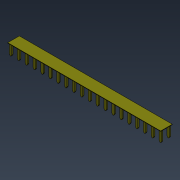
# Autodesk Inventor part: SSW-120-01-F-D_pin
Saved by Autodesk Inventor 2022.1 (Build 261234020, 234B)
## iProperties
Created: 2015-08-09
Part Number: SSW-120-01-F-D_pin
Catalog Web Link: www.cadenas.de
Description: SSW Series Pin-SSW Series - (2,54 mm) .100" Surface Mount Terminal & Through-Hole .025" Square Post Socket
Vendor: SAMTEC
Document SubType Name: Modeling
Designer: PARTuser1
Manufacturer: SAMTEC
Mass: 0.0669125 g
Surface Area: 7.06347 cm^2
Volume: 0.0669125 cm^3
Density: 1 g/cm^3
Material: Allgemein
Appearance: PSOLRGB-255-255-0
Category: PARTsolutions
Company: SAMTEC
PSOL_IDENT_0: {$CADENAS_DATA\23d-libs\samtec\modelling\ssw\parts\ssw_pin.prj},220 {VTYP=3D},{NB=SSW-120-01-F-D_pin
PSOL_IDENT_1: },{LINA=SSW-120-01-F-D_pin},{NN=SSW Series Pin},{DATE=19.06.2015 09:33:41},{GEOMDATE=19.06.2015 09:3
PSOL_IDENT_2: 3:00},{VERSION=},{LINEID=10},{LINESUBID=-1},{WBVAR=POS,LS,PLOPT,ROW,TOPT,POLOPT,LLOPT}  {NB=SSW-120-
PSOL_IDENT_3: 01-F-D_pin},{LINA=SSW-120-01-F-D_pin},{KT=DUMMY},{PN=SSW-120-01-F-D},{SERIES=SSW},{POS=20},{POSATOF=
PSOL_IDENT_4: 20},{LS=01},{LSALG= '01','-01','02','-02','03','-03','04','-04','06','-06','21','-21','22','-22','23'
PSOL_IDENT_5: ,'-23','24','-24' },{PLOPT=F},{PLOPTALG= 'G','-G - Gold, 20micro\" Au / 50micro\" Ni Min on Contact,
PSOL_IDENT_6: 3micro\" Au / 50micro\" Ni Min on Tail','S','-S - Selective, 30micro\" Au / 50micro\" Ni Min on Con
PSOL_IDENT_7: tact, Matte Tin Tail','H','-H - Heavy Gold 30micro\" Au / 50micro\" Ni Min on Contact, 3micro\" Au /
PSOL_IDENT_8: 50micro\" Ni Min on Tail' ,'F','-F - Flash Selective, 3micro\" Au / 50micro\" Ni Min on Contact, Ma
PSOL_IDENT_9: tte Tin Tail','STL','-STL - Selective, 30micro\" Au / 50micro\" Ni Min on Contact Area, Tin/Lead (90
PSOL_IDENT_10: /10 +/-5%) Tail','SM','-SM - Selective, 30micro\" Au / 50micro\" Ni Min on Contact, Matte Tin Tail','
PSOL_IDENT_11: FM','-FM - Flash Selective, 3micro\" Au / 50micro\" Ni Min on Contact, Matte Tin Tail','L','-L - Lig
PSOL_IDENT_12: ht Selective, 10micro\" Au / 50micro\" Ni Min on Contact Area, Matte Tin Tail','T','-T - Matte Tin C
PSOL_IDENT_13: ontact and Tail','E','-E - 50micro\" Extra Heavy Gold in Contact Area, 3micro\" Gold on Tail','TL','
PSOL_IDENT_14: -TL - Tin/Lead (90/10 ± 5%) Contact and Tail','TM','-TM - Matte Tin Contact and Tail' },{ROW=D},{ROW
PSOL_IDENT_15: ALG= 'S','-S - Single','D','-D - Double','T','-T - Triple', 'P','-P - Single Notched','Q','-Q - Trip
PSOL_IDENT_16: le with only Outer 2 Rows Filled' },{TOPT=},{TOPTALG= '','Straight' },{TOPTPN=},{POLOPT=},{POLOPTALG=
PSOL_IDENT_17: '','Not Selected','001','001','002','002','003','003','004','004','005','005','006','006','007','00
PSOL_IDENT_18: 7','008','008','009','009','010','010','011','011','012','012','013','013','014','014','015','015','
PSOL_IDENT_19: 016','016','017','017','018','018','019','019','020','020','021','021','022','022','023','023','024'
PSOL_IDENT_20: ,'024','025','025','026','026','027','027','028','028','029','029','030','030','031','031','032','03
PSOL_IDENT_21: 2','033','033','034','034','035','035','036','036','037','037','038','038','039','039','040','040' }
PSOL_IDENT_22: ,{POLOPTMAX=480},{POLOPTMAX2='001','001','002','002','003','003','004','004','005','005','006','006'
PSOL_IDENT_23: ,'007','007','008','008','009','009','010','010','011','011','012','012','013','013','014','014','01
PSOL_IDENT_24: 5','015','016','016','017','017','018','018','019','019','020','020','021','021','022','022','023','
PSOL_IDENT_25: 023','024','024','025','025','026','026','027','027','028','028','029','029','030','030','031','031'
PSOL_IDENT_26: ,'032','032','033','033','034','034','035','035','036','036','037','037','038','038','039','039','04
PSOL_IDENT_27: 0','040'},{POLARIZE='001','001','002','002','003','003','004','004','005','005','006','006','007','0
PSOL_IDENT_28: 07','008','008','009','009','010','010','011','011','012','012','013','013','014','014','015','015','
PSOL_IDENT_29: 016','016','017','017','018','018','019','019','020','020','021','021','022','022','023','023','024'
PSOL_IDENT_30: ,'024','025','025','026','026','027','027','028','028','029','029','030','030','031','031','032','03
PSOL_IDENT_31: 2','033','033','034','034','035','035','036','036','037','037','038','038','039','039','040','040','
PSOL_IDENT_32: 041','041','042','042','043','043','044','044','045','045','046','046','047','047','048','048','049'
PSOL_IDENT_33: ,'049','050','050','051','051','052','052','053','053','054','054','055','055','056','056','057','05
PSOL_IDENT_34: 7','058','058','059','059','060','060','061','061','062','062','063','063','064','064','065','065','
PSOL_IDENT_35: 066','066','067','067','068','068','069','069','070','070','071','071','072','072','073','073','074'
PSOL_IDENT_36: ,'074','075','075','076','076','077','077','078','078','079','079','080','080','081','081','082','08
PSOL_IDENT_37: 2','083','083','084','084','085','085','086','086','087','087','088','088','089','089','090','090','
PSOL_IDENT_38: 091','091','092','092','093','093','094','094','095','095','096','096','097','097','098','098','099'
PSOL_IDENT_39: ,'099','100','100','101','101','102','102','103','103','104','104','105','105','106','106','107','10
PSOL_IDENT_40: 7','108','108','109','109','110','110','111','111','112','112','113','113','114','114','115','115','
PSOL_IDENT_41: 116','116','117','117','118','118','119','119','120','120','121','121','122','122','123','123','124'
PSOL_IDENT_42: ,'124','125','125','126','126','127','127','128','128','129','129','130','130','131','131','132','13
PSOL_IDENT_43: 2','133','133','134','134','135','135','136','136','137','137','138','138','139','139','140','140','
PSOL_IDENT_44: 141','141','142','142','143','143','144','144','145','145','146','146','147','147','148','148','149'
PSOL_IDENT_45: ,'149','150','150'},{POLOPTPN=},{LLOPT=},{LLOPTALG= '','Not Selected','LL','-LL - Locking Lead' },{L
PSOL_IDENT_46: LOPTPN=},{B=0.104},{C=0.000},{R=2.020},{OEN=2}
NN: SSW Series Pin
NT: SSW Series - (2,54 mm) .100" Surface Mount Terminal & Through-Hole .025" Square Post Socket
NB: SSW-120-01-F-D_pin
NBSYN: $PN._pin
LINA: SSW-120-01-F-D_pin
SERIES: SSW
POS: -20
LS: -01
PLOPT: -F - Flash Selective, 3micro" Au / 50micro" Ni Min on Contact, Matte Tin Tail
ROW: -D - Double
TOPT: Straight
POLOPT: Not Selected
LLOPT: Not Selected
SUPPLIER: SAMTEC
ARTICLENO: SSW-120-01-F-D_pin
BOMINFO: SSW-120-01-F-D_pin
CREATOR: CADENAS GmbH
Title: SSW-120-01-F-D_pin
Author: Cadenas PARTsolutions
Comments: SSW Series - (2,54 mm) .100" Surface Mount Terminal & Through-Hole .025" Square Post Socket
Autodesk Inventor part; units mm, degrees
sketch "Sketch_2" plane through (0, 0, 0) normal (1, 0, 0) x (0, 1, 0)
  line L0 (3.6576, 1.4732) -> (0, 1.4732)
  line L1 (0, 1.4732) -> (0, 1.0668)
  line L2 (0, 1.0668) -> (3.5306, 1.0668)
  line L3 (3.5306, 1.0668) -> (3.5306, -1.0668)
  line L4 (3.5306, -1.0668) -> (0, -1.0668)
  line L5 (0, -1.0668) -> (0, -1.4732)
  line L6 (0, -1.4732) -> (3.6576, -1.4732)
  line L7 (3.6576, -1.4732) -> (3.6576, 1.4732)
  constraints: 16 end point
extrude "Extrusion1" add sketch "Sketch_2" along normal mid plane 49.3014
sketch "Sketch_13" plane through (0, 3.5306, 0) normal (0, 1, 0) x (1, 0, 0)
  line L0 (-24.6507, 1.8796) -> (-24.6507, -1.8796)
  line L1 (-24.6507, -1.8796) -> (24.6507, -1.8796)
  line L2 (24.6507, -1.8796) -> (24.6507, 1.8796)
  line L3 (24.6507, 1.8796) -> (-24.6507, 1.8796)
  constraints: 8 end point
extrude "Extrusion2" add sketch "Sketch_13" along normal blind 0.127
sketch "Sketch_8" plane through (0, 0, 0) normal (0, 0, 1) x (1, 0, 0)
  line L0 (-26.2763, -21.8694) -> (99.9363, -21.8694)
  line L1 (99.9363, -21.8694) -> (99.9363, 3.5306)
  line L2 (99.9363, 3.5306) -> (98.1837, 3.5306)
  line L3 (98.1837, 3.5306) -> (98.1837, -8.89)
  line L4 (98.1837, -8.89) -> (97.3963, -8.89)
  line L5 (97.3963, -8.89) -> (97.3963, 3.5306)
  line L6 (97.3963, 3.5306) -> (95.6437, 3.5306)
  line L7 (95.6437, 3.5306) -> (95.6437, -8.89)
  line L8 (95.6437, -8.89) -> (94.8563, -8.89)
  line L9 (94.8563, -8.89) -> (94.8563, 3.5306)
  line L10 (94.8563, 3.5306) -> (93.1037, 3.5306)
  line L11 (93.1037, 3.5306) -> (93.1037, -8.89)
  line L12 (93.1037, -8.89) -> (92.3163, -8.89)
  line L13 (92.3163, -8.89) -> (92.3163, 3.5306)
  line L14 (92.3163, 3.5306) -> (90.5637, 3.5306)
  line L15 (90.5637, 3.5306) -> (90.5637, -8.89)
  line L16 (90.5637, -8.89) -> (89.7763, -8.89)
  line L17 (89.7763, -8.89) -> (89.7763, 3.5306)
  line L18 (89.7763, 3.5306) -> (88.0237, 3.5306)
  line L19 (88.0237, 3.5306) -> (88.0237, -8.89)
  line L20 (88.0237, -8.89) -> (87.2363, -8.89)
  line L21 (87.2363, -8.89) -> (87.2363, 3.5306)
  line L22 (87.2363, 3.5306) -> (85.4837, 3.5306)
  line L23 (85.4837, 3.5306) -> (85.4837, -8.89)
  line L24 (85.4837, -8.89) -> (84.6963, -8.89)
  line L25 (84.6963, -8.89) -> (84.6963, 3.5306)
  line L26 (84.6963, 3.5306) -> (82.9437, 3.5306)
  line L27 (82.9437, 3.5306) -> (82.9437, -8.89)
  line L28 (82.9437, -8.89) -> (82.1563, -8.89)
  line L29 (82.1563, -8.89) -> (82.1563, 3.5306)
  line L30 (82.1563, 3.5306) -> (80.4037, 3.5306)
  line L31 (80.4037, 3.5306) -> (80.4037, -8.89)
  line L32 (80.4037, -8.89) -> (79.6163, -8.89)
  line L33 (79.6163, -8.89) -> (79.6163, 3.5306)
  line L34 (79.6163, 3.5306) -> (77.8637, 3.5306)
  line L35 (77.8637, 3.5306) -> (77.8637, -8.89)
  line L36 (77.8637, -8.89) -> (77.0763, -8.89)
  line L37 (77.0763, -8.89) -> (77.0763, 3.5306)
  line L38 (77.0763, 3.5306) -> (75.3237, 3.5306)
  line L39 (75.3237, 3.5306) -> (75.3237, -8.89)
  line L40 (75.3237, -8.89) -> (74.5363, -8.89)
  line L41 (74.5363, -8.89) -> (74.5363, 3.5306)
  line L42 (74.5363, 3.5306) -> (72.7837, 3.5306)
  line L43 (72.7837, 3.5306) -> (72.7837, -8.89)
  line L44 (72.7837, -8.89) -> (71.9963, -8.89)
  line L45 (71.9963, -8.89) -> (71.9963, 3.5306)
  line L46 (71.9963, 3.5306) -> (70.2437, 3.5306)
  line L47 (70.2437, 3.5306) -> (70.2437, -8.89)
  line L48 (70.2437, -8.89) -> (69.4563, -8.89)
  line L49 (69.4563, -8.89) -> (69.4563, 3.5306)
  line L50 (69.4563, 3.5306) -> (67.7037, 3.5306)
  line L51 (67.7037, 3.5306) -> (67.7037, -8.89)
  line L52 (67.7037, -8.89) -> (66.9163, -8.89)
  line L53 (66.9163, -8.89) -> (66.9163, 3.5306)
  line L54 (66.9163, 3.5306) -> (65.1637, 3.5306)
  line L55 (65.1637, 3.5306) -> (65.1637, -8.89)
  line L56 (65.1637, -8.89) -> (64.3763, -8.89)
  line L57 (64.3763, -8.89) -> (64.3763, 3.5306)
  line L58 (64.3763, 3.5306) -> (62.6237, 3.5306)
  line L59 (62.6237, 3.5306) -> (62.6237, -8.89)
  line L60 (62.6237, -8.89) -> (61.8363, -8.89)
  line L61 (61.8363, -8.89) -> (61.8363, 3.5306)
  line L62 (61.8363, 3.5306) -> (60.0837, 3.5306)
  line L63 (60.0837, 3.5306) -> (60.0837, -8.89)
  line L64 (60.0837, -8.89) -> (59.2963, -8.89)
  line L65 (59.2963, -8.89) -> (59.2963, 3.5306)
  line L66 (59.2963, 3.5306) -> (57.5437, 3.5306)
  line L67 (57.5437, 3.5306) -> (57.5437, -8.89)
  line L68 (57.5437, -8.89) -> (56.7563, -8.89)
  line L69 (56.7563, -8.89) -> (56.7563, 3.5306)
  line L70 (56.7563, 3.5306) -> (55.0037, 3.5306)
  line L71 (55.0037, 3.5306) -> (55.0037, -8.89)
  line L72 (55.0037, -8.89) -> (54.2163, -8.89)
  line L73 (54.2163, -8.89) -> (54.2163, 3.5306)
  line L74 (54.2163, 3.5306) -> (52.4637, 3.5306)
  line L75 (52.4637, 3.5306) -> (52.4637, -8.89)
  line L76 (52.4637, -8.89) -> (51.6763, -8.89)
  line L77 (51.6763, -8.89) -> (51.6763, 3.5306)
  line L78 (51.6763, 3.5306) -> (49.9237, 3.5306)
  line L79 (49.9237, 3.5306) -> (49.9237, -8.89)
  line L80 (49.9237, -8.89) -> (49.1363, -8.89)
  line L81 (49.1363, -8.89) -> (49.1363, 3.5306)
  line L82 (49.1363, 3.5306) -> (47.3837, 3.5306)
  line L83 (47.3837, 3.5306) -> (47.3837, -8.89)
  line L84 (47.3837, -8.89) -> (46.5963, -8.89)
  line L85 (46.5963, -8.89) -> (46.5963, 3.5306)
  line L86 (46.5963, 3.5306) -> (44.8437, 3.5306)
  line L87 (44.8437, 3.5306) -> (44.8437, -8.89)
  line L88 (44.8437, -8.89) -> (44.0563, -8.89)
  line L89 (44.0563, -8.89) -> (44.0563, 3.5306)
  line L90 (44.0563, 3.5306) -> (42.3037, 3.5306)
  line L91 (42.3037, 3.5306) -> (42.3037, -8.89)
  line L92 (42.3037, -8.89) -> (41.5163, -8.89)
  line L93 (41.5163, -8.89) -> (41.5163, 3.5306)
  line L94 (41.5163, 3.5306) -> (39.7637, 3.5306)
  line L95 (39.7637, 3.5306) -> (39.7637, -8.89)
  line L96 (39.7637, -8.89) -> (38.9763, -8.89)
  line L97 (38.9763, -8.89) -> (38.9763, 3.5306)
  line L98 (38.9763, 3.5306) -> (37.2237, 3.5306)
  line L99 (37.2237, 3.5306) -> (37.2237, -8.89)
  line L100 (37.2237, -8.89) -> (36.4363, -8.89)
  line L101 (36.4363, -8.89) -> (36.4363, 3.5306)
  line L102 (36.4363, 3.5306) -> (34.6837, 3.5306)
  line L103 (34.6837, 3.5306) -> (34.6837, -8.89)
  line L104 (34.6837, -8.89) -> (33.8963, -8.89)
  line L105 (33.8963, -8.89) -> (33.8963, 3.5306)
  line L106 (33.8963, 3.5306) -> (32.1437, 3.5306)
  line L107 (32.1437, 3.5306) -> (32.1437, -8.89)
  line L108 (32.1437, -8.89) -> (31.3563, -8.89)
  line L109 (31.3563, -8.89) -> (31.3563, 3.5306)
  line L110 (31.3563, 3.5306) -> (29.6037, 3.5306)
  line L111 (29.6037, 3.5306) -> (29.6037, -8.89)
  line L112 (29.6037, -8.89) -> (28.8163, -8.89)
  line L113 (28.8163, -8.89) -> (28.8163, 3.5306)
  line L114 (28.8163, 3.5306) -> (27.0637, 3.5306)
  line L115 (27.0637, 3.5306) -> (27.0637, -8.89)
  line L116 (27.0637, -8.89) -> (26.2763, -8.89)
  line L117 (26.2763, -8.89) -> (26.2763, 3.5306)
  line L118 (26.2763, 3.5306) -> (24.5237, 3.5306)
  line L119 (24.5237, 3.5306) -> (24.5237, -8.89)
  line L120 (24.5237, -8.89) -> (23.7363, -8.89)
  line L121 (23.7363, -8.89) -> (23.7363, 3.5306)
  line L122 (23.7363, 3.5306) -> (21.9837, 3.5306)
  line L123 (21.9837, 3.5306) -> (21.9837, -8.89)
  line L124 (21.9837, -8.89) -> (21.1963, -8.89)
  line L125 (21.1963, -8.89) -> (21.1963, 3.5306)
  line L126 (21.1963, 3.5306) -> (19.4437, 3.5306)
  line L127 (19.4437, 3.5306) -> (19.4437, -8.89)
  line L128 (19.4437, -8.89) -> (18.6563, -8.89)
  line L129 (18.6563, -8.89) -> (18.6563, 3.5306)
  line L130 (18.6563, 3.5306) -> (16.9037, 3.5306)
  line L131 (16.9037, 3.5306) -> (16.9037, -8.89)
  line L132 (16.9037, -8.89) -> (16.1163, -8.89)
  line L133 (16.1163, -8.89) -> (16.1163, 3.5306)
  line L134 (16.1163, 3.5306) -> (14.3637, 3.5306)
  line L135 (14.3637, 3.5306) -> (14.3637, -8.89)
  line L136 (14.3637, -8.89) -> (13.5763, -8.89)
  line L137 (13.5763, -8.89) -> (13.5763, 3.5306)
  line L138 (13.5763, 3.5306) -> (11.8237, 3.5306)
  line L139 (11.8237, 3.5306) -> (11.8237, -8.89)
  line L140 (11.8237, -8.89) -> (11.0363, -8.89)
  line L141 (11.0363, -8.89) -> (11.0363, 3.5306)
  line L142 (11.0363, 3.5306) -> (9.2837, 3.5306)
  line L143 (9.2837, 3.5306) -> (9.2837, -8.89)
  line L144 (9.2837, -8.89) -> (8.4963, -8.89)
  line L145 (8.4963, -8.89) -> (8.4963, 3.5306)
  line L146 (8.4963, 3.5306) -> (6.7437, 3.5306)
  line L147 (6.7437, 3.5306) -> (6.7437, -8.89)
  line L148 (6.7437, -8.89) -> (5.9563, -8.89)
  line L149 (5.9563, -8.89) -> (5.9563, 3.5306)
  line L150 (5.9563, 3.5306) -> (4.2037, 3.5306)
  line L151 (4.2037, 3.5306) -> (4.2037, -8.89)
  line L152 (4.2037, -8.89) -> (3.4163, -8.89)
  line L153 (3.4163, -8.89) -> (3.4163, 3.5306)
  line L154 (3.4163, 3.5306) -> (1.6637, 3.5306)
  line L155 (1.6637, 3.5306) -> (1.6637, -8.89)
  line L156 (1.6637, -8.89) -> (0.8763, -8.89)
  line L157 (0.8763, -8.89) -> (0.8763, 3.5306)
  line L158 (0.8763, 3.5306) -> (-0.8763, 3.5306)
  line L159 (-0.8763, 3.5306) -> (-0.8763, -8.89)
  line L160 (-0.8763, -8.89) -> (-1.6637, -8.89)
  line L161 (-1.6637, -8.89) -> (-1.6637, 3.5306)
  line L162 (-1.6637, 3.5306) -> (-3.4163, 3.5306)
  line L163 (-3.4163, 3.5306) -> (-3.4163, -8.89)
  line L164 (-3.4163, -8.89) -> (-4.2037, -8.89)
  line L165 (-4.2037, -8.89) -> (-4.2037, 3.5306)
  line L166 (-4.2037, 3.5306) -> (-5.9563, 3.5306)
  line L167 (-5.9563, 3.5306) -> (-5.9563, -8.89)
  line L168 (-5.9563, -8.89) -> (-6.7437, -8.89)
  line L169 (-6.7437, -8.89) -> (-6.7437, 3.5306)
  line L170 (-6.7437, 3.5306) -> (-8.4963, 3.5306)
  line L171 (-8.4963, 3.5306) -> (-8.4963, -8.89)
  line L172 (-8.4963, -8.89) -> (-9.2837, -8.89)
  line L173 (-9.2837, -8.89) -> (-9.2837, 3.5306)
  line L174 (-9.2837, 3.5306) -> (-11.0363, 3.5306)
  line L175 (-11.0363, 3.5306) -> (-11.0363, -8.89)
  line L176 (-11.0363, -8.89) -> (-11.8237, -8.89)
  line L177 (-11.8237, -8.89) -> (-11.8237, 3.5306)
  line L178 (-11.8237, 3.5306) -> (-13.5763, 3.5306)
  line L179 (-13.5763, 3.5306) -> (-13.5763, -8.89)
  line L180 (-13.5763, -8.89) -> (-14.3637, -8.89)
  line L181 (-14.3637, -8.89) -> (-14.3637, 3.5306)
  line L182 (-14.3637, 3.5306) -> (-16.1163, 3.5306)
  line L183 (-16.1163, 3.5306) -> (-16.1163, -8.89)
  line L184 (-16.1163, -8.89) -> (-16.9037, -8.89)
  line L185 (-16.9037, -8.89) -> (-16.9037, 3.5306)
  line L186 (-16.9037, 3.5306) -> (-18.6563, 3.5306)
  line L187 (-18.6563, 3.5306) -> (-18.6563, -8.89)
  line L188 (-18.6563, -8.89) -> (-19.4437, -8.89)
  line L189 (-19.4437, -8.89) -> (-19.4437, 3.5306)
  line L190 (-19.4437, 3.5306) -> (-21.1963, 3.5306)
  line L191 (-21.1963, 3.5306) -> (-21.1963, -8.89)
  line L192 (-21.1963, -8.89) -> (-21.9837, -8.89)
  line L193 (-21.9837, -8.89) -> (-21.9837, 3.5306)
  line L194 (-21.9837, 3.5306) -> (-23.7363, 3.5306)
  line L195 (-23.7363, 3.5306) -> (-23.7363, -8.89)
  line L196 (-23.7363, -8.89) -> (-24.5237, -8.89)
  line L197 (-24.5237, -8.89) -> (-24.5237, 3.5306)
  line L198 (-24.5237, 3.5306) -> (-26.2763, 3.5306)
  line L199 (-26.2763, 3.5306) -> (-26.2763, -21.8694)
  constraints: 400 end point
extrude "Extrusion3" cut sketch "Sketch_8" along normal mid plane 50.8
sketch "Sketch_6" plane through (0, 0, 0) normal (0, 0, 1) x (1, 0, 0)
  line L0 (-24.5237, 0.4399) -> (-24.5237, -2.54)
  line L1 (-24.5237, -2.54) -> (24.5237, -2.54)
  line L2 (24.5237, -2.54) -> (24.5237, 0.4399)
  line L3 (24.5237, 0.4399) -> (24.2697, 0)
  line L4 (24.2697, 0) -> (23.9903, 0)
  line L5 (23.9903, 0) -> (23.7363, 0.4399)
  line L6 (23.7363, 0.4399) -> (23.7363, -2.032)
  line L7 (23.7363, -2.032) -> (21.9837, -2.032)
  line L8 (21.9837, -2.032) -> (21.9837, 0.4399)
  line L9 (21.9837, 0.4399) -> (21.7297, 0)
  line L10 (21.7297, 0) -> (21.4503, 0)
  line L11 (21.4503, 0) -> (21.1963, 0.4399)
  line L12 (21.1963, 0.4399) -> (21.1963, -2.032)
  line L13 (21.1963, -2.032) -> (19.4437, -2.032)
  line L14 (19.4437, -2.032) -> (19.4437, 0.4399)
  line L15 (19.4437, 0.4399) -> (19.1897, 0)
  line L16 (19.1897, 0) -> (18.9103, 0)
  line L17 (18.9103, 0) -> (18.6563, 0.4399)
  line L18 (18.6563, 0.4399) -> (18.6563, -2.032)
  line L19 (18.6563, -2.032) -> (16.9037, -2.032)
  line L20 (16.9037, -2.032) -> (16.9037, 0.4399)
  line L21 (16.9037, 0.4399) -> (16.6497, 0)
  line L22 (16.6497, 0) -> (16.3703, 0)
  line L23 (16.3703, 0) -> (16.1163, 0.4399)
  line L24 (16.1163, 0.4399) -> (16.1163, -2.032)
  line L25 (16.1163, -2.032) -> (14.3637, -2.032)
  line L26 (14.3637, -2.032) -> (14.3637, 0.4399)
  line L27 (14.3637, 0.4399) -> (14.1097, 0)
  line L28 (14.1097, 0) -> (13.8303, 0)
  line L29 (13.8303, 0) -> (13.5763, 0.4399)
  line L30 (13.5763, 0.4399) -> (13.5763, -2.032)
  line L31 (13.5763, -2.032) -> (11.8237, -2.032)
  line L32 (11.8237, -2.032) -> (11.8237, 0.4399)
  line L33 (11.8237, 0.4399) -> (11.5697, 0)
  line L34 (11.5697, 0) -> (11.2903, 0)
  line L35 (11.2903, 0) -> (11.0363, 0.4399)
  line L36 (11.0363, 0.4399) -> (11.0363, -2.032)
  line L37 (11.0363, -2.032) -> (9.2837, -2.032)
  line L38 (9.2837, -2.032) -> (9.2837, 0.4399)
  line L39 (9.2837, 0.4399) -> (9.0297, 0)
  line L40 (9.0297, 0) -> (8.7503, 0)
  line L41 (8.7503, 0) -> (8.4963, 0.4399)
  line L42 (8.4963, 0.4399) -> (8.4963, -2.032)
  line L43 (8.4963, -2.032) -> (6.7437, -2.032)
  line L44 (6.7437, -2.032) -> (6.7437, 0.4399)
  line L45 (6.7437, 0.4399) -> (6.4897, 0)
  line L46 (6.4897, 0) -> (6.2103, 0)
  line L47 (6.2103, 0) -> (5.9563, 0.4399)
  line L48 (5.9563, 0.4399) -> (5.9563, -2.032)
  line L49 (5.9563, -2.032) -> (4.2037, -2.032)
  line L50 (4.2037, -2.032) -> (4.2037, 0.4399)
  line L51 (4.2037, 0.4399) -> (3.9497, 0)
  line L52 (3.9497, 0) -> (3.6703, 0)
  line L53 (3.6703, 0) -> (3.4163, 0.4399)
  line L54 (3.4163, 0.4399) -> (3.4163, -2.032)
  line L55 (3.4163, -2.032) -> (1.6637, -2.032)
  line L56 (1.6637, -2.032) -> (1.6637, 0.4399)
  line L57 (1.6637, 0.4399) -> (1.4097, 0)
  line L58 (1.4097, 0) -> (1.1303, 0)
  line L59 (1.1303, 0) -> (0.8763, 0.4399)
  line L60 (0.8763, 0.4399) -> (0.8763, -2.032)
  line L61 (0.8763, -2.032) -> (-0.8763, -2.032)
  line L62 (-0.8763, -2.032) -> (-0.8763, 0.4399)
  line L63 (-0.8763, 0.4399) -> (-1.1303, 0)
  line L64 (-1.1303, 0) -> (-1.4097, 0)
  line L65 (-1.4097, 0) -> (-1.6637, 0.4399)
  line L66 (-1.6637, 0.4399) -> (-1.6637, -2.032)
  line L67 (-1.6637, -2.032) -> (-3.4163, -2.032)
  line L68 (-3.4163, -2.032) -> (-3.4163, 0.4399)
  line L69 (-3.4163, 0.4399) -> (-3.6703, 0)
  line L70 (-3.6703, 0) -> (-3.9497, 0)
  line L71 (-3.9497, 0) -> (-4.2037, 0.4399)
  line L72 (-4.2037, 0.4399) -> (-4.2037, -2.032)
  line L73 (-4.2037, -2.032) -> (-5.9563, -2.032)
  line L74 (-5.9563, -2.032) -> (-5.9563, 0.4399)
  line L75 (-5.9563, 0.4399) -> (-6.2103, 0)
  line L76 (-6.2103, 0) -> (-6.4897, 0)
  line L77 (-6.4897, 0) -> (-6.7437, 0.4399)
  line L78 (-6.7437, 0.4399) -> (-6.7437, -2.032)
  line L79 (-6.7437, -2.032) -> (-8.4963, -2.032)
  line L80 (-8.4963, -2.032) -> (-8.4963, 0.4399)
  line L81 (-8.4963, 0.4399) -> (-8.7503, 0)
  line L82 (-8.7503, 0) -> (-9.0297, 0)
  line L83 (-9.0297, 0) -> (-9.2837, 0.4399)
  line L84 (-9.2837, 0.4399) -> (-9.2837, -2.032)
  line L85 (-9.2837, -2.032) -> (-11.0363, -2.032)
  line L86 (-11.0363, -2.032) -> (-11.0363, 0.4399)
  line L87 (-11.0363, 0.4399) -> (-11.2903, 0)
  line L88 (-11.2903, 0) -> (-11.5697, 0)
  line L89 (-11.5697, 0) -> (-11.8237, 0.4399)
  line L90 (-11.8237, 0.4399) -> (-11.8237, -2.032)
  line L91 (-11.8237, -2.032) -> (-13.5763, -2.032)
  line L92 (-13.5763, -2.032) -> (-13.5763, 0.4399)
  line L93 (-13.5763, 0.4399) -> (-13.8303, 0)
  line L94 (-13.8303, 0) -> (-14.1097, 0)
  line L95 (-14.1097, 0) -> (-14.3637, 0.4399)
  line L96 (-14.3637, 0.4399) -> (-14.3637, -2.032)
  line L97 (-14.3637, -2.032) -> (-16.1163, -2.032)
  line L98 (-16.1163, -2.032) -> (-16.1163, 0.4399)
  line L99 (-16.1163, 0.4399) -> (-16.3703, 0)
  line L100 (-16.3703, 0) -> (-16.6497, 0)
  line L101 (-16.6497, 0) -> (-16.9037, 0.4399)
  line L102 (-16.9037, 0.4399) -> (-16.9037, -2.032)
  line L103 (-16.9037, -2.032) -> (-18.6563, -2.032)
  line L104 (-18.6563, -2.032) -> (-18.6563, 0.4399)
  line L105 (-18.6563, 0.4399) -> (-18.9103, 0)
  line L106 (-18.9103, 0) -> (-19.1897, 0)
  line L107 (-19.1897, 0) -> (-19.4437, 0.4399)
  line L108 (-19.4437, 0.4399) -> (-19.4437, -2.032)
  line L109 (-19.4437, -2.032) -> (-21.1963, -2.032)
  line L110 (-21.1963, -2.032) -> (-21.1963, 0.4399)
  line L111 (-21.1963, 0.4399) -> (-21.4503, 0)
  line L112 (-21.4503, 0) -> (-21.7297, 0)
  line L113 (-21.7297, 0) -> (-21.9837, 0.4399)
  line L114 (-21.9837, 0.4399) -> (-21.9837, -2.032)
  line L115 (-21.9837, -2.032) -> (-23.7363, -2.032)
  line L116 (-23.7363, -2.032) -> (-23.7363, 0.4399)
  line L117 (-23.7363, 0.4399) -> (-23.9903, 0)
  line L118 (-23.9903, 0) -> (-24.2697, 0)
  line L119 (-24.2697, 0) -> (-24.5237, 0.4399)
  constraints: 240 end point
extrude "Extrusion4" cut sketch "Sketch_6" along normal mid plane 25.4
ref_plane "pin_XY" through (0, 2.6416, 0) normal (0, -1, 0) x (1, 0, 0)
ref_plane "pin_YZ" through (0, 2.6416, 0) normal (1, 0, 0) x (0, 0, 1)
ref_plane "pin_ZX" through (0, 2.6416, 0) normal (0, 0, 1) x (0, -1, 0)
body "Solid1"
